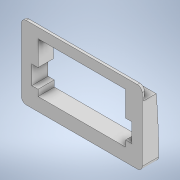
# Autodesk Inventor part: electricalCoverGasket02
Saved by Autodesk Inventor 2021.1 (Build 251245000, 245)
## iProperties
Created: 2020-08-29
Part Number: electricalCoverGasket02
Material: Generic
Document SubType Name: Modeling
Designer: robst
Density: 1 g/cm^3
Appearance: Default
Author: robst
Autodesk Inventor part; units mm, degrees
ref_plane "YZ Plane" through (0, 0, 0) normal (1, 0, 0) x (0, 1, 0)
ref_plane "XZ Plane" through (0, 0, 0) normal (0, 1, 0) x (-1, 0, 0)
sketch "Sketch1" plane through (0, 0, 0) normal (1, 0, 0) x (0, 1, 0)
  line L0 (0, 0) -> (0, 12.7)
  line L1 (0, 0) -> (-101.6, 0) construction
  arc A0 (-101.6, 0) -> (0, 0) centre (-50.8, 556.4861) ccw
  line L2 (-50.8, -2.3139) -> (-50.8, 0) construction
  line L3 (0, 12.7) -> (101.6, 12.7) construction
  arc A1 (0, 12.7) -> (101.6, 12.7) centre (50.8, 569.1861) ccw
  line L4 (12.7, 14.2265) -> (-61.5442, 14.2265)
  line L5 (-61.5442, 14.2265) -> (-61.5442, -2.2106)
  line L6 (12.7, 14.2265) -> (12.7, 11.6865)
  dimension "d5" = 558.8
  dimension "d6" = 101.6
  dimension "d7" = 558.8
  dimension "d24" = 12.7
  dimension "d26" = 74.2442
  dimension "d29" = 2.54
  dimension "d50" = 12.7
  constraints: 14 end point, 7 point on circle, 3 horizontal, 2 centre point, 2 perpendicular, 1 midpoint, 1 vertical
  measures "d5" radius of A0
  measures "d6" distance of L0.end L3.end
  measures "d7" radius of A1
  measures "d24" distance of L0.start L0.end
  measures "d26" distance of L4.start L4.end
  measures "d29" distance of L4.start L6.end
  measures "d50" distance from line of L6 L0.start
extrude "Extrusion3" add sketch "Sketch1" along normal mid plane 122.428
sketch "Sketch5" plane through (0, 0, 0) normal (0, 0, 1) x (1, 0, 0)
  line L0 (-61.214, 12.7) -> (61.214, 12.7) projected
  line L1 (-61.214, 0) -> (61.214, 0) projected
  line L2 (61.214, 0) -> (61.214, 12.7)
  line L3 (-61.214, 12.7) -> (-61.214, 0)
  line L4 (61.214, 7.62) -> (-61.214, 7.62) construction
  line L5 (-61.214, -61.5442) -> (-61.214, 12.7) construction
  line L6 (21.5694, 3.81) -> (21.5694, 10.5284)
  line L7 (21.5694, 10.5284) -> (24.1259, 10.5284)
  line L8 (24.1259, 10.5284) -> (24.1259, 11.43)
  line L9 (24.1259, 11.43) -> (18.0002, 11.43)
  line L10 (18.0002, 11.43) -> (18.0002, 10.5284)
  line L11 (18.0002, 10.5284) -> (20.5567, 10.5284)
  line L12 (20.5567, 10.5284) -> (20.5567, 3.81)
  line L13 (20.5567, 3.81) -> (21.5694, 3.81)
  spline S0 degree 2 poles (11.8314, 10.5593) (11.3991, 10.053) (10.9175, 8.571) (10.9175, 7.62) knots 0 0 0 1 2 2 2
  spline S1 degree 2 poles (10.9175, 7.62) (10.9175, 6.6937) (11.3868, 5.1932) (11.8314, 4.6869) knots 0 0 0 1 2 2 2
  spline S2 degree 2 poles (11.8314, 4.6869) (12.3007, 4.1558) (13.5419, 3.6494) (14.289, 3.6494) knots 0 0 0 1 2 2 2
  spline S3 degree 2 poles (14.289, 3.6494) (15.0609, 3.6494) (16.2959, 4.1743) (16.7467, 4.6869) knots 0 0 0 1 2 2 2
  spline S4 degree 2 poles (16.7467, 4.6869) (17.1851, 5.1932) (17.6544, 6.6814) (17.6544, 7.62) knots 0 0 0 1 2 2 2
  spline S5 degree 2 poles (17.6544, 7.62) (17.6544, 8.5771) (17.179, 10.0344) (16.7405, 10.5593) knots 0 0 0 1 2 2 2
  spline S6 degree 2 poles (16.7405, 10.5593) (16.2959, 11.0657) (15.0547, 11.5906) (14.289, 11.5906) knots 0 0 0 1 2 2 2
  spline S7 degree 2 poles (14.289, 11.5906) (13.511, 11.5906) (12.2636, 11.0471) (11.8314, 10.5593) knots 0 0 0 1 2 2 2
  spline S8 degree 2 poles (11.9734, 7.62) (11.9734, 8.3734) (12.3007, 9.5404) (12.5971, 9.9233) knots 0 0 0 1 2 2 2
  spline S9 degree 2 poles (12.5971, 9.9233) (12.8997, 10.3185) (13.7518, 10.7137) (14.2829, 10.7137) knots 0 0 0 1 2 2 2
  spline S10 degree 2 poles (14.2829, 10.7137) (14.8324, 10.7137) (15.6599, 10.3308) (15.9748, 9.9233) knots 0 0 0 1 2 2 2
  spline S11 degree 2 poles (15.9748, 9.9233) (16.2774, 9.5343) (16.5985, 8.361) (16.5985, 7.62) knots 0 0 0 1 2 2 2
  spline S12 degree 2 poles (16.5985, 7.62) (16.5985, 6.1195) (15.3388, 4.5263) (14.2829, 4.5263) knots 0 0 0 1 2 2 2
  spline S13 degree 2 poles (14.2829, 4.5263) (13.2269, 4.5263) (11.9734, 6.1195) (11.9734, 7.62) knots 0 0 0 1 2 2 2
  spline S14 degree 2 poles (4.9894, 9.1329) (4.9894, 8.6389) (5.3414, 7.7497) (5.6563, 7.4409) knots 0 0 0 1 2 2 2
  spline S15 degree 2 poles (5.6563, 7.4409) (6.0515, 7.0519) (7.1198, 6.6505) (7.9349, 6.6505) knots 0 0 0 1 2 2 2
  line L14 (7.9349, 6.6505) -> (8.7933, 6.6505)
  line L15 (8.7933, 6.6505) -> (8.7933, 3.81)
  line L16 (8.7933, 3.81) -> (9.806, 3.81)
  line L17 (9.806, 3.81) -> (9.806, 11.43)
  line L18 (9.806, 11.43) -> (7.8917, 11.43)
  spline S16 degree 2 poles (7.8917, 11.43) (7.2124, 11.43) (6.2615, 11.2077) (5.8972, 10.9545) knots 0 0 0 1 2 2 2
  spline S17 degree 2 poles (5.8972, 10.9545) (5.4711, 10.6643) (4.9894, 9.7689) (4.9894, 9.1329) knots 0 0 0 1 2 2 2
  spline S18 degree 2 poles (6.0454, 9.102) (6.0454, 9.4972) (6.3171, 10.0777) (6.5949, 10.2629) knots 0 0 0 1 2 2 2
  spline S19 degree 2 poles (6.5949, 10.2629) (6.8358, 10.4235) (7.478, 10.5531) (7.9535, 10.5531) knots 0 0 0 1 2 2 2
  line L19 (7.9535, 10.5531) -> (8.7933, 10.5531)
  line L20 (8.7933, 10.5531) -> (8.7933, 7.515)
  line L21 (8.7933, 7.515) -> (8.1017, 7.515)
  spline S20 degree 2 poles (8.1017, 7.515) (7.4841, 7.515) (6.7246, 7.7126) (6.4776, 7.972) knots 0 0 0 1 2 2 2
  spline S21 degree 2 poles (6.4776, 7.972) (6.2491, 8.2005) (6.0454, 8.7377) (6.0454, 9.102) knots 0 0 0 1 2 2 2
  line L22 (1.0745, 11.7696) -> (4.057, 2.1551)
  line L23 (4.057, 2.1551) -> (4.9215, 2.1551)
  line L24 (4.9215, 2.1551) -> (1.9513, 11.7696)
  line L25 (1.9513, 11.7696) -> (1.0745, 11.7696)
  spline S22 degree 2 poles (-5.15, 6.1503) (-5.15, 5.5822) (-4.7177, 4.7116) (-4.3596, 4.4275) knots 0 0 0 1 2 2 2
  spline S23 degree 2 poles (-4.3596, 4.4275) (-3.9273, 4.0941) (-2.9455, 3.81) (-2.1674, 3.81) knots 0 0 0 1 2 2 2
  line L26 (-2.1674, 3.81) -> (0.0185, 3.81)
  line L27 (0.0185, 3.81) -> (0.0185, 11.43)
  line L28 (0.0185, 11.43) -> (-2.0007, 11.43)
  spline S24 degree 2 poles (-2.0007, 11.43) (-2.8158, 11.43) (-3.6309, 11.325) (-4.0014, 11.1212) knots 0 0 0 1 2 2 2
  spline S25 degree 2 poles (-4.0014, 11.1212) (-4.4152, 10.9051) (-4.7918, 10.195) (-4.7918, 9.7133) knots 0 0 0 1 2 2 2
  spline S26 degree 2 poles (-4.7918, 9.7133) (-4.7918, 9.1761) (-4.2237, 8.324) (-3.7235, 8.0831) knots 0 0 0 1 2 2 2
  line L29 (-3.7235, 8.0831) -> (-3.7235, 8.0461)
  spline S27 degree 2 poles (-3.7235, 8.0461) (-4.4028, 7.8608) (-5.15, 6.879) (-5.15, 6.1503) knots 0 0 0 1 2 2 2
  spline S28 degree 2 poles (-4.0941, 6.1071) (-4.0941, 6.5394) (-3.8471, 7.0951) (-3.4765, 7.2927) knots 0 0 0 1 2 2 2
  spline S29 degree 2 poles (-3.4765, 7.2927) (-3.2357, 7.4162) (-2.6676, 7.4903) (-2.1427, 7.4903) knots 0 0 0 1 2 2 2
  line L30 (-2.1427, 7.4903) -> (-0.9942, 7.4903)
  line L31 (-0.9942, 7.4903) -> (-0.9942, 4.6745)
  line L32 (-0.9942, 4.6745) -> (-1.8155, 4.6745)
  spline S30 degree 2 poles (-1.8155, 4.6745) (-2.4824, 4.6745) (-3.2481, 4.798) (-3.5445, 4.9956) knots 0 0 0 1 2 2 2
  spline S31 degree 2 poles (-3.5445, 4.9956) (-3.8285, 5.1994) (-4.0941, 5.7057) (-4.0941, 6.1071) knots 0 0 0 1 2 2 2
  spline S32 degree 2 poles (-3.7359, 9.5713) (-3.7359, 9.843) (-3.5506, 10.2506) (-3.3469, 10.3679) knots 0 0 0 1 2 2 2
  spline S33 degree 2 poles (-3.3469, 10.3679) (-3.0999, 10.5037) (-2.5009, 10.5655) (-1.9637, 10.5655) knots 0 0 0 1 2 2 2
  line L33 (-1.9637, 10.5655) -> (-0.9942, 10.5655)
  line L34 (-0.9942, 10.5655) -> (-0.9942, 8.3363)
  line L35 (-0.9942, 8.3363) -> (-2.1427, 8.3363)
  spline S34 degree 2 poles (-2.1427, 8.3363) (-2.6182, 8.3363) (-3.069, 8.4351) (-3.3098, 8.5895) knots 0 0 0 1 2 2 2
  spline S35 degree 2 poles (-3.3098, 8.5895) (-3.5445, 8.7377) (-3.7359, 9.2132) (-3.7359, 9.5713) knots 0 0 0 1 2 2 2
  line L36 (-5.3352, 3.81) -> (-7.9041, 11.43)
  line L37 (-7.9041, 11.43) -> (-9.1514, 11.43)
  line L38 (-9.1514, 11.43) -> (-11.7202, 3.81)
  line L39 (-11.7202, 3.81) -> (-10.6519, 3.81)
  line L40 (-10.6519, 3.81) -> (-9.9603, 5.9404)
  line L41 (-9.9603, 5.9404) -> (-7.0519, 5.9404)
  line L42 (-7.0519, 5.9404) -> (-6.3603, 3.81)
  line L43 (-6.3603, 3.81) -> (-5.3352, 3.81)
  line L44 (-9.6825, 6.8049) -> (-8.503, 10.3926)
  line L45 (-8.503, 10.3926) -> (-7.3298, 6.8049)
  line L46 (-7.3298, 6.8049) -> (-9.6825, 6.8049)
  spline S36 degree 2 poles (-15.5179, 3.6741) (-14.7769, 3.6741) (-13.5233, 4.1743) (-13.0664, 4.6745) knots 0 0 0 1 2 2 2
  spline S37 degree 2 poles (-13.0664, 4.6745) (-12.6094, 5.1685) (-12.1093, 6.6505) (-12.1093, 7.6138) knots 0 0 0 1 2 2 2
  spline S38 degree 2 poles (-12.1093, 7.6138) (-12.1093, 8.571) (-12.5971, 9.9912) (-13.0602, 10.5161) knots 0 0 0 1 2 2 2
  spline S39 degree 2 poles (-13.0602, 10.5161) (-13.5172, 11.0286) (-14.7645, 11.5659) (-15.5364, 11.5659) knots 0 0 0 1 2 2 2
  spline S40 degree 2 poles (-15.5364, 11.5659) (-15.9193, 11.5659) (-16.5923, 11.4547) (-16.8764, 11.3682) knots 0 0 0 1 2 2 2
  spline S41 degree 2 poles (-16.8764, 11.3682) (-17.1234, 11.288) (-17.6359, 11.0595) (-17.8891, 10.9236) knots 0 0 0 1 2 2 2
  line L47 (-17.8891, 10.9236) -> (-17.8891, 9.701)
  line L48 (-17.8891, 9.701) -> (-17.8088, 9.701)
  spline S42 degree 2 poles (-17.8088, 9.701) (-17.673, 9.8245) (-17.2531, 10.1703) (-16.9505, 10.337) knots 0 0 0 1 2 2 2
  spline S43 degree 2 poles (-16.9505, 10.337) (-16.6603, 10.4976) (-15.9748, 10.7013) (-15.5302, 10.7013) knots 0 0 0 1 2 2 2
  spline S44 degree 2 poles (-15.5302, 10.7013) (-15.0424, 10.7013) (-14.1717, 10.3) (-13.8444, 9.9171) knots 0 0 0 1 2 2 2
  spline S45 degree 2 poles (-13.8444, 9.9171) (-13.5233, 9.5281) (-13.1652, 8.3487) (-13.1652, 7.6138) knots 0 0 0 1 2 2 2
  spline S46 degree 2 poles (-13.1652, 7.6138) (-13.1652, 6.8296) (-13.5419, 5.6996) (-13.8691, 5.3105) knots 0 0 0 1 2 2 2
  spline S47 degree 2 poles (-13.8691, 5.3105) (-14.1902, 4.9339) (-15.0486, 4.551) (-15.5302, 4.551) knots 0 0 0 1 2 2 2
  spline S48 degree 2 poles (-15.5302, 4.551) (-15.9687, 4.551) (-16.7158, 4.7671) (-17.0061, 4.9277) knots 0 0 0 1 2 2 2
  spline S49 degree 2 poles (-17.0061, 4.9277) (-17.2839, 5.0882) (-17.6977, 5.4217) (-17.815, 5.539) knots 0 0 0 1 2 2 2
  line L49 (-17.815, 5.539) -> (-17.8891, 5.539)
  line L50 (-17.8891, 5.539) -> (-17.8891, 4.3287)
  spline S50 degree 2 poles (-17.8891, 4.3287) (-17.6359, 4.2114) (-17.1913, 3.9953) (-16.8764, 3.8965) knots 0 0 0 1 2 2 2
  spline S51 degree 2 poles (-16.8764, 3.8965) (-16.5429, 3.7853) (-15.9748, 3.6741) (-15.5179, 3.6741) knots 0 0 0 1 2 2 2
  line L51 (-24.3914, 3.81) -> (-23.0761, 3.81)
  line L52 (-23.0761, 3.81) -> (-20.2912, 7.3545)
  line L53 (-20.2912, 7.3545) -> (-19.8466, 6.8543)
  line L54 (-19.8466, 6.8543) -> (-19.8466, 3.81)
  line L55 (-19.8466, 3.81) -> (-18.8339, 3.81)
  line L56 (-18.8339, 3.81) -> (-18.8339, 11.43)
  line L57 (-18.8339, 11.43) -> (-19.8466, 11.43)
  line L58 (-19.8466, 11.43) -> (-19.8466, 7.9288)
  line L59 (-19.8466, 7.9288) -> (-22.9712, 11.43)
  line L60 (-22.9712, 11.43) -> (-24.2062, 11.43)
  line L61 (-24.2062, 11.43) -> (-21.0507, 8.0276)
  line L62 (-21.0507, 8.0276) -> (-24.3914, 3.81)
  point P0 (0, 0)
  dimension "d41" = 5.08
  constraints: 6 end point, 1 horizontal
  measures "d41" distance between parallel lines of L4 L0
emboss "Emboss3" sketch "Sketch5" operation cut depth 1.016 direction (0, 0, -1) wrap yes faces at (20.4047, 11.2878, 11.7848) contours L13 L12 L11 L10 L9 L8 L7 L6 | S7 S6 S5 S4 S3 S2 S1 S0 | S17 S16 L18 L17 L16 L15 L14 S15 S14 | L25 L24 L23 L22 | S27 L29 S26 S25 S24 L28 L27 L26 S23 S22 | L43 L42 L41 L40 L39 L38 L37 L36 | S51 S50 L50 L49 S49 S48 S47 S46 S45 S44 S43 S42 L48 L47 S41 S40 S39 S38 S37 S36 | L62 L61 L60 L59 L58 L57 L56 L55 L54 L53 L52 L51
ref_plane "Work Plane3" through (0, -50.8, -2.3139) normal (0, 0, 1) x (1, 0, 0)
sketch "Sketch8" plane through (-61.214, -61.5442, 14.2265) normal (0, 0, 1) x (1, 0, 0)
  line L0 (122.428, 61.5442) -> (0, 61.5442) projected
  line L1 (61.214, 61.5442) -> (61.214, 0) construction
  line L2 (0, 0) -> (122.428, 0) construction
  line L3 (16.764, 13.335) -> (105.664, 13.335)
  line L4 (105.664, 13.335) -> (105.664, 64.135)
  line L5 (105.664, 64.135) -> (16.764, 64.135)
  line L6 (16.764, 64.135) -> (16.764, 13.335)
  line L7 (16.764, 13.335) -> (105.664, 64.135) construction
  line L8 (105.664, 13.335) -> (16.764, 64.135) construction
  point P0 (61.214, 38.735)
  dimension "d36" = 50.8
  dimension "d37" = 88.9
  dimension "d38" = 13.335
  constraints: 14 end point, 3 midpoint, 2 parallel, 2 perpendicular, 1 point on line
  measures "d36" distance of L5.end L3.start
  measures "d37" distance between parallel lines of L4 L6
  measures "d38" distance between parallel lines of L2 L3
extrude "Extrusion4" cut sketch "Sketch8" against normal through all
sketch "Sketch9" plane through (0, -50.8, -2.3139) normal (0, 0, 1) x (1, 0, 0)
  line L0 (-61.214, -10.7442) -> (61.214, -10.7442) projected
  line L1 (-44.45, 2.5908) -> (44.45, 2.5908) projected
  line L2 (-44.45, 2.5908) -> (-44.45, 53.3908) construction
  line L3 (-44.45, 2.5908) -> (-44.45, -10.7442) construction
  line L4 (-61.214, -10.7442) -> (61.214, -10.7442) construction
  line L5 (44.45, 2.5908) -> (-44.45, 2.5908) construction
  line L6 (44.45, 2.5908) -> (44.45, -10.7442) construction
  line L7 (44.45, -4.0767) -> (-44.45, -4.0767) construction
  spline S0 degree 2 poles (45.9809, -8.673) (47.5802, -8.673) (49.3381, -6.8791) (49.3381, -5.2222) knots 0 0 0 1 2 2 2
  spline S1 degree 2 poles (49.3381, -5.2222) (49.3381, -3.594) (47.6307, -1.6633) (46.2547, -1.6633) knots 0 0 0 1 2 2 2
  spline S2 degree 2 poles (46.2547, -1.6633) (45.6351, -1.6633) (44.6769, -2.0235) (44.3239, -2.4053) knots 0 0 0 1 2 2 2
  spline S3 degree 2 poles (44.3239, -2.4053) (43.9637, -2.7871) (43.5819, -3.8894) (43.5819, -4.6891) knots 0 0 0 1 2 2 2
  line L8 (43.5819, -4.6891) -> (43.5819, -5.3014)
  line L9 (43.5819, -5.3014) -> (48.1998, -5.3014)
  spline S4 degree 2 poles (48.1998, -5.3014) (48.1998, -6.4613) (47.0327, -7.6932) (45.9953, -7.6932) knots 0 0 0 1 2 2 2
  spline S5 degree 2 poles (45.9953, -7.6932) (45.6279, -7.6932) (44.9147, -7.5275) (44.6265, -7.3978) knots 0 0 0 1 2 2 2
  spline S6 degree 2 poles (44.6265, -7.3978) (44.3239, -7.2538) (43.9061, -7.0016) (43.7692, -6.8863) knots 0 0 0 1 2 2 2
  line L10 (43.7692, -6.8863) -> (43.7044, -6.8863)
  line L11 (43.7044, -6.8863) -> (43.7044, -8.1111)
  spline S7 degree 2 poles (43.7044, -8.1111) (43.8989, -8.1903) (44.4896, -8.4208) (44.7202, -8.4857) knots 0 0 0 1 2 2 2
  spline S8 degree 2 poles (44.7202, -8.4857) (45.0443, -8.5793) (45.5775, -8.673) (45.9809, -8.673) knots 0 0 0 1 2 2 2
  spline S9 degree 2 poles (44.6769, -4.4441) (44.6913, -3.9902) (44.8787, -3.3275) (45.0588, -3.1041) knots 0 0 0 1 2 2 2
  spline S10 degree 2 poles (45.0588, -3.1041) (45.2533, -2.852) (45.8656, -2.5854) (46.3195, -2.5854) knots 0 0 0 1 2 2 2
  spline S11 degree 2 poles (46.3195, -2.5854) (46.7662, -2.5854) (47.3929, -2.852) (47.6523, -3.1113) knots 0 0 0 1 2 2 2
  spline S12 degree 2 poles (47.6523, -3.1113) (47.9044, -3.3779) (48.1638, -4.0191) (48.1998, -4.4441) knots 0 0 0 1 2 2 2
  line L12 (48.1998, -4.4441) -> (44.6769, -4.4441)
  spline S13 degree 2 poles (38.8847, -8.6802) (39.7493, -8.6802) (41.2117, -8.0967) (41.7448, -7.5131) knots 0 0 0 1 2 2 2
  spline S14 degree 2 poles (41.7448, -7.5131) (42.2779, -6.9368) (42.8615, -5.2078) (42.8615, -4.0839) knots 0 0 0 1 2 2 2
  spline S15 degree 2 poles (42.8615, -4.0839) (42.8615, -2.9673) (42.2923, -1.3103) (41.752, -0.6979) knots 0 0 0 1 2 2 2
  spline S16 degree 2 poles (41.752, -0.6979) (41.2189, -0.1) (39.7637, 0.5268) (38.8631, 0.5268) knots 0 0 0 1 2 2 2
  spline S17 degree 2 poles (38.8631, 0.5268) (38.4165, 0.5268) (37.6312, 0.3971) (37.2998, 0.2963) knots 0 0 0 1 2 2 2
  spline S18 degree 2 poles (37.2998, 0.2963) (37.0117, 0.2026) (36.4137, -0.064) (36.1183, -0.2224) knots 0 0 0 1 2 2 2
  line L13 (36.1183, -0.2224) -> (36.1183, -1.6489)
  line L14 (36.1183, -1.6489) -> (36.212, -1.6489)
  spline S19 degree 2 poles (36.212, -1.6489) (36.3705, -1.5048) (36.8604, -1.1014) (37.2134, -0.9068) knots 0 0 0 1 2 2 2
  spline S20 degree 2 poles (37.2134, -0.9068) (37.552, -0.7195) (38.3516, -0.4818) (38.8703, -0.4818) knots 0 0 0 1 2 2 2
  spline S21 degree 2 poles (38.8703, -0.4818) (39.4395, -0.4818) (40.4553, -0.9501) (40.8371, -1.3967) knots 0 0 0 1 2 2 2
  spline S22 degree 2 poles (40.8371, -1.3967) (41.2117, -1.8506) (41.6296, -3.2266) (41.6296, -4.0839) knots 0 0 0 1 2 2 2
  spline S23 degree 2 poles (41.6296, -4.0839) (41.6296, -4.9988) (41.1901, -6.3172) (40.8083, -6.7711) knots 0 0 0 1 2 2 2
  spline S24 degree 2 poles (40.8083, -6.7711) (40.4337, -7.2105) (39.4323, -7.6572) (38.8703, -7.6572) knots 0 0 0 1 2 2 2
  spline S25 degree 2 poles (38.8703, -7.6572) (38.3588, -7.6572) (37.4871, -7.405) (37.1485, -7.2177) knots 0 0 0 1 2 2 2
  spline S26 degree 2 poles (37.1485, -7.2177) (36.8243, -7.0304) (36.3417, -6.6414) (36.2048, -6.5045) knots 0 0 0 1 2 2 2
  line L15 (36.2048, -6.5045) -> (36.1183, -6.5045)
  line L16 (36.1183, -6.5045) -> (36.1183, -7.9165)
  spline S27 degree 2 poles (36.1183, -7.9165) (36.4137, -8.0534) (36.9324, -8.3056) (37.2998, -8.4208) knots 0 0 0 1 2 2 2
  spline S28 degree 2 poles (37.2998, -8.4208) (37.6888, -8.5505) (38.3516, -8.6802) (38.8847, -8.6802) knots 0 0 0 1 2 2 2
  spline S29 degree 2 poles (31.2915, -8.6946) (32.2353, -8.6946) (33.7986, -8.1183) (34.3605, -7.5347) knots 0 0 0 1 2 2 2
  spline S30 degree 2 poles (34.3605, -7.5347) (34.9224, -6.944) (35.5204, -5.2006) (35.5204, -4.0695) knots 0 0 0 1 2 2 2
  spline S31 degree 2 poles (35.5204, -4.0695) (35.5204, -2.9961) (34.9152, -1.2959) (34.3533, -0.6907) knots 0 0 0 1 2 2 2
  spline S32 degree 2 poles (34.3533, -0.6907) (33.813, -0.1072) (32.2281, 0.5268) (31.2843, 0.5268) knots 0 0 0 1 2 2 2
  spline S33 degree 2 poles (31.2843, 0.5268) (30.8304, 0.5268) (30.0092, 0.3971) (29.6345, 0.2818) knots 0 0 0 1 2 2 2
  spline S34 degree 2 poles (29.6345, 0.2818) (29.332, 0.1954) (28.5971, -0.1216) (28.3738, -0.2369) knots 0 0 0 1 2 2 2
  line L17 (28.3738, -0.2369) -> (28.3738, -1.6633)
  line L18 (28.3738, -1.6633) -> (28.4747, -1.6633)
  spline S35 degree 2 poles (28.4747, -1.6633) (28.698, -1.4688) (29.1663, -1.1158) (29.5985, -0.9141) knots 0 0 0 1 2 2 2
  spline S36 degree 2 poles (29.5985, -0.9141) (29.9587, -0.7339) (30.8881, -0.4962) (31.4212, -0.4962) knots 0 0 0 1 2 2 2
  spline S37 degree 2 poles (31.4212, -0.4962) (32.7035, -0.4962) (34.2885, -2.4269) (34.2885, -4.0335) knots 0 0 0 1 2 2 2
  spline S38 degree 2 poles (34.2885, -4.0335) (34.2885, -4.9268) (33.8706, -6.2668) (33.4744, -6.7279) knots 0 0 0 1 2 2 2
  spline S39 degree 2 poles (33.4744, -6.7279) (33.0926, -7.1889) (32.0119, -7.6716) (31.3347, -7.6716) knots 0 0 0 1 2 2 2
  spline S40 degree 2 poles (31.3347, -7.6716) (30.8376, -7.6716) (29.8435, -7.5275) (29.5049, -7.3834) knots 0 0 0 1 2 2 2
  line L19 (29.5049, -7.3834) -> (29.5049, -5.0853)
  line L20 (29.5049, -5.0853) -> (31.5653, -5.0853)
  line L21 (31.5653, -5.0853) -> (31.5653, -4.0479)
  line L22 (31.5653, -4.0479) -> (28.3378, -4.0479)
  line L23 (28.3378, -4.0479) -> (28.3378, -7.931)
  spline S41 degree 2 poles (28.3378, -7.931) (28.5611, -8.0318) (29.3248, -8.3416) (29.6489, -8.4352) knots 0 0 0 1 2 2 2
  spline S42 degree 2 poles (29.6489, -8.4352) (30.0884, -8.5649) (30.7944, -8.6946) (31.2915, -8.6946) knots 0 0 0 1 2 2 2
  spline S43 degree 2 poles (21.573, -4.0767) (21.573, -6.4685) (22.9634, -8.709) (24.4115, -8.709) knots 0 0 0 1 2 2 2
  spline S44 degree 2 poles (24.4115, -8.709) (25.8811, -8.709) (27.2571, -6.4253) (27.2571, -4.0839) knots 0 0 0 1 2 2 2
  spline S45 degree 2 poles (27.2571, -4.0839) (27.2571, -1.6777) (25.8667, 0.5484) (24.4115, 0.5484) knots 0 0 0 1 2 2 2
  spline S46 degree 2 poles (24.4115, 0.5484) (22.949, 0.5484) (21.573, -1.7569) (21.573, -4.0767) knots 0 0 0 1 2 2 2
  spline S47 degree 2 poles (23.1003, -6.7855) (22.9274, -6.346) (22.7833, -4.9916) (22.7833, -4.0767) knots 0 0 0 1 2 2 2
  spline S48 degree 2 poles (22.7833, -4.0767) (22.7833, -3.1618) (22.9274, -1.8146) (23.1075, -1.3607) knots 0 0 0 1 2 2 2
  spline S49 degree 2 poles (23.1075, -1.3607) (23.2876, -0.9068) (23.9144, -0.4386) (24.4115, -0.4386) knots 0 0 0 1 2 2 2
  spline S50 degree 2 poles (24.4115, -0.4386) (24.9086, -0.4386) (25.5497, -0.9068) (25.7371, -1.3751) knots 0 0 0 1 2 2 2
  spline S51 degree 2 poles (25.7371, -1.3751) (25.9172, -1.829) (26.0468, -3.2122) (26.0468, -4.0839) knots 0 0 0 1 2 2 2
  spline S52 degree 2 poles (26.0468, -4.0839) (26.0468, -5.0205) (25.9316, -6.274) (25.7443, -6.7639) knots 0 0 0 1 2 2 2
  spline S53 degree 2 poles (25.7443, -6.7639) (25.5714, -7.2249) (24.9302, -7.722) (24.4115, -7.722) knots 0 0 0 1 2 2 2
  spline S54 degree 2 poles (24.4115, -7.722) (23.9216, -7.722) (23.2804, -7.2538) (23.1003, -6.7855) knots 0 0 0 1 2 2 2
  line L24 (14.9523, -8.5217) -> (20.4348, -8.5217)
  line L25 (20.4348, -8.5217) -> (20.4348, -7.261)
  spline S55 degree 2 poles (20.4348, -7.261) (19.844, -6.7062) (18.7922, -5.676) (18.2879, -5.1213) knots 0 0 0 1 2 2 2
  spline S56 degree 2 poles (18.2879, -5.1213) (17.2721, -4.0047) (16.5301, -2.6647) (16.5301, -1.9515) knots 0 0 0 1 2 2 2
  spline S57 degree 2 poles (16.5301, -1.9515) (16.5301, -1.5768) (16.7606, -1.0149) (16.9695, -0.8348) knots 0 0 0 1 2 2 2
  spline S58 degree 2 poles (16.9695, -0.8348) (17.1784, -0.6547) (17.726, -0.4746) (18.0574, -0.4746) knots 0 0 0 1 2 2 2
  spline S59 degree 2 poles (18.0574, -0.4746) (18.3743, -0.4746) (19.0227, -0.6331) (19.3181, -0.7556) knots 0 0 0 1 2 2 2
  spline S60 degree 2 poles (19.3181, -0.7556) (19.5702, -0.8564) (20.0385, -1.1446) (20.1826, -1.2454) knots 0 0 0 1 2 2 2
  line L26 (20.1826, -1.2454) -> (20.2474, -1.2454)
  line L27 (20.2474, -1.2454) -> (20.2474, 0.0225)
  spline S61 degree 2 poles (20.2474, 0.0225) (19.88, 0.2026) (18.5617, 0.5556) (17.9709, 0.5556) knots 0 0 0 1 2 2 2
  spline S62 degree 2 poles (17.9709, 0.5556) (16.7246, 0.5556) (15.3198, -0.7628) (15.3198, -1.8866) knots 0 0 0 1 2 2 2
  spline S63 degree 2 poles (15.3198, -1.8866) (15.3198, -2.4125) (15.5647, -3.2914) (15.7808, -3.6661) knots 0 0 0 1 2 2 2
  spline S64 degree 2 poles (15.7808, -3.6661) (15.997, -4.0551) (16.6237, -4.8187) (16.9695, -5.1861) knots 0 0 0 1 2 2 2
  spline S65 degree 2 poles (16.9695, -5.1861) (17.5315, -5.7985) (18.9075, -7.1097) (19.3181, -7.4915) knots 0 0 0 1 2 2 2
  line L28 (19.3181, -7.4915) -> (14.9523, -7.4915)
  line L29 (14.9523, -7.4915) -> (14.9523, -8.5217)
  spline S66 degree 2 poles (4.1893, -5.006) (4.1893, -6.6774) (5.7814, -8.6514) (6.9989, -8.6514) knots 0 0 0 1 2 2 2
  spline S67 degree 2 poles (6.9989, -8.6514) (7.496, -8.6514) (8.2596, -8.4208) (8.6559, -8.1831) knots 0 0 0 1 2 2 2
  line L30 (8.6559, -8.1831) -> (8.6559, -10.9783)
  line L31 (8.6559, -10.9783) -> (9.7797, -10.9783)
  line L32 (9.7797, -10.9783) -> (9.7797, -1.8506)
  line L33 (9.7797, -1.8506) -> (8.6559, -1.8506)
  line L34 (8.6559, -1.8506) -> (8.6559, -2.5494)
  spline S68 degree 2 poles (8.6559, -2.5494) (8.238, -2.1676) (7.215, -1.6633) (6.6171, -1.6633) knots 0 0 0 1 2 2 2
  spline S69 degree 2 poles (6.6171, -1.6633) (5.4716, -1.6633) (4.1893, -3.4788) (4.1893, -5.006) knots 0 0 0 1 2 2 2
  spline S70 degree 2 poles (5.3491, -5.1357) (5.3491, -3.9902) (6.0768, -2.7295) (6.8908, -2.7295) knots 0 0 0 1 2 2 2
  spline S71 degree 2 poles (6.8908, -2.7295) (7.3663, -2.7295) (8.2596, -3.1546) (8.6559, -3.486) knots 0 0 0 1 2 2 2
  line L35 (8.6559, -3.486) -> (8.6559, -7.2754)
  spline S72 degree 2 poles (8.6559, -7.2754) (8.2164, -7.4843) (7.5896, -7.6428) (7.1862, -7.6428) knots 0 0 0 1 2 2 2
  spline S73 degree 2 poles (7.1862, -7.6428) (6.3145, -7.6428) (5.3491, -6.3604) (5.3491, -5.1357) knots 0 0 0 1 2 2 2
  line L36 (-3.5121, 0.3683) -> (-0.4503, -8.5217)
  line L37 (-0.4503, -8.5217) -> (0.8249, -8.5217)
  line L38 (0.8249, -8.5217) -> (3.8867, 0.3683)
  line L39 (3.8867, 0.3683) -> (2.6187, 0.3683)
  line L40 (2.6187, 0.3683) -> (0.1549, -7.016)
  line L41 (0.1549, -7.016) -> (-2.3089, 0.3683)
  line L42 (-2.3089, 0.3683) -> (-3.5121, 0.3683)
  spline S74 degree 2 poles (-9.7437, -4.0767) (-9.7437, -6.4685) (-8.3533, -8.709) (-6.9052, -8.709) knots 0 0 0 1 2 2 2
  spline S75 degree 2 poles (-6.9052, -8.709) (-5.4356, -8.709) (-4.0596, -6.4253) (-4.0596, -4.0839) knots 0 0 0 1 2 2 2
  spline S76 degree 2 poles (-4.0596, -4.0839) (-4.0596, -1.6777) (-5.45, 0.5484) (-6.9052, 0.5484) knots 0 0 0 1 2 2 2
  spline S77 degree 2 poles (-6.9052, 0.5484) (-8.3677, 0.5484) (-9.7437, -1.7569) (-9.7437, -4.0767) knots 0 0 0 1 2 2 2
  spline S78 degree 2 poles (-8.2164, -6.7855) (-8.3893, -6.346) (-8.5334, -4.9916) (-8.5334, -4.0767) knots 0 0 0 1 2 2 2
  spline S79 degree 2 poles (-8.5334, -4.0767) (-8.5334, -3.1618) (-8.3893, -1.8146) (-8.2092, -1.3607) knots 0 0 0 1 2 2 2
  spline S80 degree 2 poles (-8.2092, -1.3607) (-8.0291, -0.9068) (-7.4023, -0.4386) (-6.9052, -0.4386) knots 0 0 0 1 2 2 2
  spline S81 degree 2 poles (-6.9052, -0.4386) (-6.4081, -0.4386) (-5.767, -0.9068) (-5.5797, -1.3751) knots 0 0 0 1 2 2 2
  spline S82 degree 2 poles (-5.5797, -1.3751) (-5.3996, -1.829) (-5.2699, -3.2122) (-5.2699, -4.0839) knots 0 0 0 1 2 2 2
  spline S83 degree 2 poles (-5.2699, -4.0839) (-5.2699, -5.0205) (-5.3851, -6.274) (-5.5725, -6.7639) knots 0 0 0 1 2 2 2
  spline S84 degree 2 poles (-5.5725, -6.7639) (-5.7454, -7.2249) (-6.3865, -7.722) (-6.9052, -7.722) knots 0 0 0 1 2 2 2
  spline S85 degree 2 poles (-6.9052, -7.722) (-7.3951, -7.722) (-8.0363, -7.2538) (-8.2164, -6.7855) knots 0 0 0 1 2 2 2
  spline S86 degree 2 poles (-13.281, -0.4746) (-12.9568, -0.4746) (-12.3156, -0.6331) (-12.0058, -0.7556) knots 0 0 0 1 2 2 2
  spline S87 degree 2 poles (-12.0058, -0.7556) (-11.7177, -0.878) (-11.2926, -1.1374) (-11.1269, -1.2526) knots 0 0 0 1 2 2 2
  line L43 (-11.1269, -1.2526) -> (-11.0549, -1.2526)
  line L44 (-11.0549, -1.2526) -> (-11.0549, 0.0081)
  spline S88 degree 2 poles (-11.0549, 0.0081) (-11.4439, 0.217) (-12.7767, 0.5556) (-13.3746, 0.5556) knots 0 0 0 1 2 2 2
  spline S89 degree 2 poles (-13.3746, 0.5556) (-13.9798, 0.5556) (-14.8803, 0.3107) (-15.2477, 0.0513) knots 0 0 0 1 2 2 2
  spline S90 degree 2 poles (-15.2477, 0.0513) (-15.6367, -0.2296) (-16.0402, -1.0437) (-16.0402, -1.5912) knots 0 0 0 1 2 2 2
  spline S91 degree 2 poles (-16.0402, -1.5912) (-16.0402, -2.3261) (-15.0748, -3.4355) (-14.3976, -3.5796) knots 0 0 0 1 2 2 2
  line L45 (-14.3976, -3.5796) -> (-14.3976, -3.6661)
  spline S92 degree 2 poles (-14.3976, -3.6661) (-14.6786, -3.7237) (-15.3198, -3.983) (-15.5935, -4.2424) knots 0 0 0 1 2 2 2
  spline S93 degree 2 poles (-15.5935, -4.2424) (-15.8673, -4.4945) (-16.2131, -5.3014) (-16.2131, -5.885) knots 0 0 0 1 2 2 2
  spline S94 degree 2 poles (-16.2131, -5.885) (-16.2131, -6.4829) (-15.8024, -7.4987) (-15.4278, -7.8877) knots 0 0 0 1 2 2 2
  spline S95 degree 2 poles (-15.4278, -7.8877) (-15.0388, -8.2912) (-13.9365, -8.709) (-13.2377, -8.709) knots 0 0 0 1 2 2 2
  spline S96 degree 2 poles (-13.2377, -8.709) (-12.5677, -8.709) (-11.2566, -8.3848) (-10.8099, -8.1615) knots 0 0 0 1 2 2 2
  line L46 (-10.8099, -8.1615) -> (-10.8099, -6.9008)
  line L47 (-10.8099, -6.9008) -> (-10.8964, -6.9008)
  spline S97 degree 2 poles (-10.8964, -6.9008) (-11.271, -7.1745) (-12.5389, -7.6788) (-13.1657, -7.6788) knots 0 0 0 1 2 2 2
  spline S98 degree 2 poles (-13.1657, -7.6788) (-13.5331, -7.6788) (-14.2679, -7.4483) (-14.5129, -7.1817) knots 0 0 0 1 2 2 2
  spline S99 degree 2 poles (-14.5129, -7.1817) (-14.7506, -6.9152) (-15.0028, -6.2812) (-15.0028, -5.7985) knots 0 0 0 1 2 2 2
  spline S100 degree 2 poles (-15.0028, -5.7985) (-15.0028, -5.3158) (-14.7218, -4.6891) (-14.4697, -4.509) knots 0 0 0 1 2 2 2
  spline S101 degree 2 poles (-14.4697, -4.509) (-14.2175, -4.3288) (-13.5331, -4.192) (-13.1297, -4.192) knots 0 0 0 1 2 2 2
  line L48 (-13.1297, -4.192) -> (-12.6254, -4.192)
  line L49 (-12.6254, -4.192) -> (-12.6254, -3.205)
  line L50 (-12.6254, -3.205) -> (-13.0216, -3.205)
  spline S102 degree 2 poles (-13.0216, -3.205) (-13.8213, -3.205) (-14.8299, -2.4413) (-14.8299, -1.7137) knots 0 0 0 1 2 2 2
  spline S103 degree 2 poles (-14.8299, -1.7137) (-14.8299, -1.3751) (-14.5705, -0.8924) (-14.3616, -0.7484) knots 0 0 0 1 2 2 2
  spline S104 degree 2 poles (-14.3616, -0.7484) (-14.1383, -0.5971) (-13.5907, -0.4746) (-13.281, -0.4746) knots 0 0 0 1 2 2 2
  spline S105 degree 2 poles (-27.6534, -5.7913) (-27.6534, -6.4541) (-27.1491, -7.4699) (-26.7312, -7.8013) knots 0 0 0 1 2 2 2
  spline S106 degree 2 poles (-26.7312, -7.8013) (-26.2269, -8.1903) (-25.0815, -8.5217) (-24.1737, -8.5217) knots 0 0 0 1 2 2 2
  line L51 (-24.1737, -8.5217) -> (-21.6234, -8.5217)
  line L52 (-21.6234, -8.5217) -> (-21.6234, 0.3683)
  line L53 (-21.6234, 0.3683) -> (-23.9792, 0.3683)
  spline S107 degree 2 poles (-23.9792, 0.3683) (-24.9302, 0.3683) (-25.8811, 0.2458) (-26.3134, 0.0081) knots 0 0 0 1 2 2 2
  spline S108 degree 2 poles (-26.3134, 0.0081) (-26.7961, -0.2441) (-27.2355, -1.0725) (-27.2355, -1.6345) knots 0 0 0 1 2 2 2
  spline S109 degree 2 poles (-27.2355, -1.6345) (-27.2355, -2.2612) (-26.5727, -3.2554) (-25.9892, -3.5364) knots 0 0 0 1 2 2 2
  line L54 (-25.9892, -3.5364) -> (-25.9892, -3.5796)
  spline S110 degree 2 poles (-25.9892, -3.5796) (-26.7817, -3.7957) (-27.6534, -4.9412) (-27.6534, -5.7913) knots 0 0 0 1 2 2 2
  spline S111 degree 2 poles (-26.4215, -5.8417) (-26.4215, -5.3374) (-26.1333, -4.6891) (-25.701, -4.4585) knots 0 0 0 1 2 2 2
  spline S112 degree 2 poles (-25.701, -4.4585) (-25.4201, -4.3144) (-24.7573, -4.228) (-24.1449, -4.228) knots 0 0 0 1 2 2 2
  line L55 (-24.1449, -4.228) -> (-22.8049, -4.228)
  line L56 (-22.8049, -4.228) -> (-22.8049, -7.5131)
  line L57 (-22.8049, -7.5131) -> (-23.7631, -7.5131)
  spline S113 degree 2 poles (-23.7631, -7.5131) (-24.5412, -7.5131) (-25.4345, -7.369) (-25.7803, -7.1385) knots 0 0 0 1 2 2 2
  spline S114 degree 2 poles (-25.7803, -7.1385) (-26.1117, -6.9008) (-26.4215, -6.31) (-26.4215, -5.8417) knots 0 0 0 1 2 2 2
  spline S115 degree 2 poles (-26.0036, -1.8002) (-26.0036, -1.4832) (-25.7875, -1.0077) (-25.5497, -0.8708) knots 0 0 0 1 2 2 2
  spline S116 degree 2 poles (-25.5497, -0.8708) (-25.2616, -0.7123) (-24.5628, -0.6403) (-23.936, -0.6403) knots 0 0 0 1 2 2 2
  line L58 (-23.936, -0.6403) -> (-22.8049, -0.6403)
  line L59 (-22.8049, -0.6403) -> (-22.8049, -3.241)
  line L60 (-22.8049, -3.241) -> (-24.1449, -3.241)
  spline S117 degree 2 poles (-24.1449, -3.241) (-24.6996, -3.241) (-25.2256, -3.1257) (-25.5065, -2.9456) knots 0 0 0 1 2 2 2
  spline S118 degree 2 poles (-25.5065, -2.9456) (-25.7803, -2.7727) (-26.0036, -2.218) (-26.0036, -1.8002) knots 0 0 0 1 2 2 2
  line L61 (-27.8695, -8.5217) -> (-30.8665, 0.3683)
  line L62 (-30.8665, 0.3683) -> (-32.3217, 0.3683)
  line L63 (-32.3217, 0.3683) -> (-35.3187, -8.5217)
  line L64 (-35.3187, -8.5217) -> (-34.0723, -8.5217)
  line L65 (-34.0723, -8.5217) -> (-33.2655, -6.0362)
  line L66 (-33.2655, -6.0362) -> (-29.8723, -6.0362)
  line L67 (-29.8723, -6.0362) -> (-29.0654, -8.5217)
  line L68 (-29.0654, -8.5217) -> (-27.8695, -8.5217)
  line L69 (-32.9413, -5.0277) -> (-31.5653, -0.842)
  line L70 (-31.5653, -0.842) -> (-30.1965, -5.0277)
  line L71 (-30.1965, -5.0277) -> (-32.9413, -5.0277)
  spline S119 degree 2 poles (-39.7492, -8.6802) (-38.8847, -8.6802) (-37.4223, -8.0967) (-36.8892, -7.5131) knots 0 0 0 1 2 2 2
  spline S120 degree 2 poles (-36.8892, -7.5131) (-36.3561, -6.9368) (-35.7725, -5.2078) (-35.7725, -4.0839) knots 0 0 0 1 2 2 2
  spline S121 degree 2 poles (-35.7725, -4.0839) (-35.7725, -2.9673) (-36.3417, -1.3103) (-36.882, -0.6979) knots 0 0 0 1 2 2 2
  spline S122 degree 2 poles (-36.882, -0.6979) (-37.4151, -0.1) (-38.8703, 0.5268) (-39.7709, 0.5268) knots 0 0 0 1 2 2 2
  spline S123 degree 2 poles (-39.7709, 0.5268) (-40.2175, 0.5268) (-41.0028, 0.3971) (-41.3342, 0.2963) knots 0 0 0 1 2 2 2
  spline S124 degree 2 poles (-41.3342, 0.2963) (-41.6223, 0.2026) (-42.2203, -0.064) (-42.5157, -0.2224) knots 0 0 0 1 2 2 2
  line L72 (-42.5157, -0.2224) -> (-42.5157, -1.6489)
  line L73 (-42.5157, -1.6489) -> (-42.422, -1.6489)
  spline S125 degree 2 poles (-42.422, -1.6489) (-42.2635, -1.5048) (-41.7736, -1.1014) (-41.4206, -0.9068) knots 0 0 0 1 2 2 2
  spline S126 degree 2 poles (-41.4206, -0.9068) (-41.082, -0.7195) (-40.2824, -0.4818) (-39.7637, -0.4818) knots 0 0 0 1 2 2 2
  spline S127 degree 2 poles (-39.7637, -0.4818) (-39.1945, -0.4818) (-38.1787, -0.9501) (-37.7969, -1.3967) knots 0 0 0 1 2 2 2
  spline S128 degree 2 poles (-37.7969, -1.3967) (-37.4223, -1.8506) (-37.0044, -3.2266) (-37.0044, -4.0839) knots 0 0 0 1 2 2 2
  spline S129 degree 2 poles (-37.0044, -4.0839) (-37.0044, -4.9988) (-37.4439, -6.3172) (-37.8257, -6.7711) knots 0 0 0 1 2 2 2
  spline S130 degree 2 poles (-37.8257, -6.7711) (-38.2003, -7.2105) (-39.2017, -7.6572) (-39.7637, -7.6572) knots 0 0 0 1 2 2 2
  spline S131 degree 2 poles (-39.7637, -7.6572) (-40.2752, -7.6572) (-41.1469, -7.405) (-41.4855, -7.2177) knots 0 0 0 1 2 2 2
  spline S132 degree 2 poles (-41.4855, -7.2177) (-41.8097, -7.0304) (-42.2923, -6.6414) (-42.4292, -6.5045) knots 0 0 0 1 2 2 2
  line L74 (-42.4292, -6.5045) -> (-42.5157, -6.5045)
  line L75 (-42.5157, -6.5045) -> (-42.5157, -7.9165)
  spline S133 degree 2 poles (-42.5157, -7.9165) (-42.2203, -8.0534) (-41.7016, -8.3056) (-41.3342, -8.4208) knots 0 0 0 1 2 2 2
  spline S134 degree 2 poles (-41.3342, -8.4208) (-40.9451, -8.5505) (-40.2824, -8.6802) (-39.7492, -8.6802) knots 0 0 0 1 2 2 2
  line L76 (-50.1017, -8.5217) -> (-48.5672, -8.5217)
  line L77 (-48.5672, -8.5217) -> (-45.3181, -4.3865)
  line L78 (-45.3181, -4.3865) -> (-44.7994, -4.97)
  line L79 (-44.7994, -4.97) -> (-44.7994, -8.5217)
  line L80 (-44.7994, -8.5217) -> (-43.6179, -8.5217)
  line L81 (-43.6179, -8.5217) -> (-43.6179, 0.3683)
  line L82 (-43.6179, 0.3683) -> (-44.7994, 0.3683)
  line L83 (-44.7994, 0.3683) -> (-44.7994, -3.7165)
  line L84 (-44.7994, -3.7165) -> (-48.4447, 0.3683)
  line L85 (-48.4447, 0.3683) -> (-49.8856, 0.3683)
  line L86 (-49.8856, 0.3683) -> (-46.2042, -3.6012)
  line L87 (-46.2042, -3.6012) -> (-50.1017, -8.5217)
  point P0 (0, 50.8)
  constraints: 6 end point, 2 midpoint, 2 perpendicular, 2 point on line, 1 horizontal
emboss "Emboss5" sketch "Sketch9" operation cut depth 1.016 direction (0, 0, -1) wrap yes faces at (-14.8167, -57.0995, -2.2784)
fillet "Fillet1" radius 4.7625 4 edges at (-61.214, 12.7, 12.9565) (-61.214, -61.5442, 6.008) (61.214, -61.5442, 6.008) (61.214, 12.7, 12.9565)
sketch "Sketch10" plane through (-56.4515, 12.7, 14.2265) normal (0, 0, 1) x (1, 0, 0)
  line L0 (12.0015, -60.9092) -> (12.0015, -10.1092) projected
  line L1 (12.0015, -10.1092) -> (100.9015, -10.1092) projected
  line L2 (100.9015, -10.1092) -> (100.9015, -60.9092) projected
  line L3 (100.9015, -60.9092) -> (12.0015, -60.9092) projected
  line L4 (12.0015, -10.1092) -> (12.0015, -12.7) construction
  line L5 (12.0015, -45.0342) -> (100.9015, -45.0342) construction
  line L6 (5.6515, -54.5592) -> (18.3515, -54.5592)
  line L7 (18.3515, -54.5592) -> (18.3515, -35.5092)
  line L8 (18.3515, -35.5092) -> (5.6515, -35.5092)
  line L9 (5.6515, -35.5092) -> (5.6515, -54.5592)
  line L10 (5.6515, -54.5592) -> (18.3515, -35.5092) construction
  line L11 (18.3515, -54.5592) -> (5.6515, -35.5092) construction
  line L12 (94.5515, -54.5592) -> (107.2515, -54.5592)
  line L13 (107.2515, -54.5592) -> (107.2515, -35.5092)
  line L14 (107.2515, -35.5092) -> (94.5515, -35.5092)
  line L15 (94.5515, -35.5092) -> (94.5515, -54.5592)
  line L16 (94.5515, -54.5592) -> (107.2515, -35.5092) construction
  line L17 (107.2515, -54.5592) -> (94.5515, -35.5092) construction
  line L18 (100.9015, -60.9092) -> (100.9015, -12.7) projected
  point P0 (56.4515, -12.7)
  point P1 (100.9015, -35.5092)
  point P2 (100.9015, -54.5592)
  point P3 (12.0015, -54.5592)
  point P4 (12.0015, -35.5092)
  dimension "d45" = 34.925
  dimension "d46" = 12.7
  dimension "d47" = 19.05
  constraints: 26 end point, 4 midpoint, 4 parallel, 4 perpendicular, 2 equal length, 2 point on line, 1 horizontal
  measures "d45" distance between parallel lines of L5 L1
  measures "d46" distance of L7.end L8.end
  measures "d47" distance of L8.end L6.start
extrude "Extrusion5" cut sketch "Sketch10" against normal through all contours L6 L9 L8 L0 | L2 L14 L13 L12
equation "\"d5\" = radiusOfCurvature"
equation "\"d6\" = sidingHeight"
equation "\"d7\" = radiusOfCurvature"
equation "\"d24\" = sidingDepth"
equation "\"d26\" = coverHeight"
equation "\"d29\" = partMinDepth"
equation "\"d50\" = topAboveEdge"
equation "\"d30\" = coverWidth"
equation "\"d41\" = topCenterLineForText"
equation "\"d32\" = textDepth"
equation "\"d36\" = insideHoleHeight"
equation "\"d37\" = insideHoleWidth"
equation "\"d42\" = textDepth"
equation "\"d44\" = filletRadiusAroundEdges"
equation "\"sidingHeight\" = 101.6"
equation "\"sidingDepth\" = 12.7"
equation "\"radiusOfCurvature\" = 558.8"
equation "\"partMinDepth\" = 2.54"
equation "\"coverHeight\" = 74.2442"
equation "\"coverWidth\" = 122.428"
equation "\"electricalPlugHeight\" = 38.1"
equation "\"insideHoleWidth\" = 88.9"
equation "\"insideHoleHeight\" = 50.8"
equation "\"textDepth\" = 1.016"
equation "\"textCenterLine\" = 6.6675"
equation "\"filletRadiusAroundEdges\" = 4.7625"
equation "\"topAboveEdge\" = 12.7"
equation "\"topCenterLineForText\" = 5.08"
body "Solid1"
body "Solid2"
